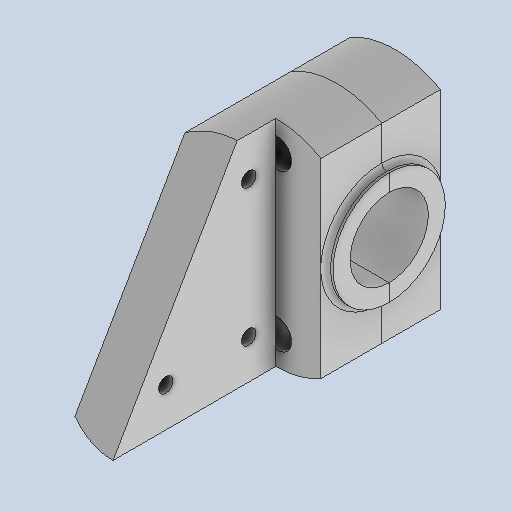
# Autodesk Inventor part: 1042
Saved by Autodesk Inventor 2025.1 (Build 291241000, 241)
## iProperties
Created: 2024-06-10
Part Number: 1042
Material: Generisch
Document SubType Name: Modeling
Designer: ffogue
Density: 1 g/cm^3
Appearance: Vorgabe
Author: ffogue
Autodesk Inventor part; units mm, degrees
note: some values were not read from the file. Chosen so that the rebuilt part matches the saved one: direction of "Bohrung4"; direction of "Bohrung11"; direction of "Bohrung12".
sketch "Skizze1" plane through (0, 0, 0) normal (0, 1, 0) x (-1, 0, 0)
  line L0 (9.25, 16.0215) -> (9.25, -23.0215)
  line L1 (-9.25, 16.0215) -> (-9.25, -23.0215)
  arc A0 (-9.25, -23.0215) -> (9.25, -23.0215) centre (0, -7) ccw
  arc A1 (9.25, 16.0215) -> (-9.25, 16.0215) centre (0, 0) ccw
  line L2 (9.25, -3.5) -> (-9.25, -3.5) construction
  line L3 (0, 18.5) -> (0, -26.5698) construction
  point P0 (0, -25.5)
  dimension "d1" = 18.5
  dimension "d2" = 44
  dimension "d3" = 18.5
  constraints: 8 end point, 6 point on circle, 2 centre point, 2 midpoint, 2 vertical, 1 coincident, 1 parallel, 1 symmetric about line, 1 other
  measures "d1" distance between parallel lines of L1 L0
  measures "d2" distance of point (0, -25.5) L3.start
  measures "d3" radius of A0
extrude "Extrusion1" add sketch "Skizze1" along normal blind 57.8
sketch "Skizze2" plane through (9.25, 0, 16.0215) normal (1, 0, 0) x (0, 0, -1)
  line L0 (0, 0) -> (-2.4785, 0) projected
  line L1 (41.5215, 0) -> (41.5215, 57.8) projected
  line L2 (0, 0) -> (39.0429, 0) projected
  line L3 (41.5215, 0) -> (39.0429, 0) projected
  line L4 (-2.4785, 0) -> (-2.4785, 57.8) projected
  line L5 (41.5215, 0) -> (-2.4785, 25.4034)
  point P0 (16.0215, 0)
  dimension "d143" = 60
  constraints: 2 end point, 1 point on line
  measures "d143" angle of L4 L5
extrude "Extrusion2" cut sketch "Skizze2" against normal up to surface (18.5 mm away)
ref_plane "Arbeitsebene1" through (0, 45.8, 0) normal (0, 1, 0) x (-1, 0, 0)
sketch "Skizze8" plane through (-9.25, 57.8, -23.0215) normal (-1, 0, 0) x (0, 0, 1)
  circle A0 centre (19.5215, -12) radius 11.5
  line L0 (0, 0) -> (39.0429, 0) projected
  point P0 (23.0215, -57.8)
  point P1 (19.5215, 0)
  dimension "d40" = 23
  dimension "d41" = 12
  constraints: 1 centre point, 1 midpoint, 1 vertical alignment
  measures "d40" diameter of A0
  measures "d41" distance from line of L0 A0.centre
extrude "Extrusion5" add sketch "Skizze8" along normal mid plane 1.5
sketch "Skizze9" plane through (9.25, 57.8, 16.0215) normal (1, 0, 0) x (0, 0, -1)
  circle A0 centre (19.5215, -12) radius 11.5
  line L0 (0, 0) -> (39.0429, 0) projected
  point P0 (16.0215, -57.8)
  point P1 (19.5215, 0)
  dimension "d44" = 23
  dimension "d45" = 12
  constraints: 1 centre point, 1 midpoint, 1 vertical alignment
  measures "d44" diameter of A0
  measures "d45" distance from line of A0.centre L0
extrude "Extrusion6" add sketch "Skizze9" along normal blind 1.5
sketch "Skizze10" plane through (10.75, 45.8, -3.5) normal (1, 0, 0) x (0, 0, -1)
  circle A0 centre (0, 0) radius 11.5 projected
  point P0 (-3.5, -45.8)
  constraints: 1 coincident
hole "Bohrung4" at (10.75, 45.8, -3.5) direction (-1, 0, 0) diameter 16 depth 20.75
ref_plane "Arbeitsebene2" through (0, 45.8, 0) normal (0, 1, 0) x (-1, 0, 0)
split_face "Trennen2"
sketch "Skizze11" plane through (0, 57.8, 0) normal (0, 1, 0) x (1, 0, 0)
  line L0 (0, 0) -> (5.4139, 0) construction
  arc A0 (-9.25, -16.0215) -> (9.25, -16.0215) centre (0, 0) ccw projected
  line L1 (0, -18.5) -> (0, 25.5) construction
  arc A1 (9.25, 23.0215) -> (-9.25, 23.0215) centre (0, 7) ccw projected
  point P0 (0, -12.5)
  point P1 (0, 19.5)
  point P2 (0, 3.5)
  dimension "d67" = 16
  dimension "d68" = 32
  constraints: 4 end point, 2 point on circle, 2 vertical alignment, 1 horizontal, 1 midpoint, 1 vertical
  measures "d67" distance of point (0, 3.5) point (0, -12.5)
  measures "d68" distance of point (0, 19.5) point (0, -12.5)
ref_plane "Arbeitsebene3" through (0, 0, 0) normal (1, 0, 0) x (0, 1, 0)
fillet "Rundung1" radius 1 2 edges at (9.25, 45.8, 8) (-9.25, 45.8, -15)
sketch "Skizze17" plane through (0, 0, 0) normal (1, 0, 0) x (0, 1, 0)
  line L0 (0, -25.5) -> (45.8, -25.5) projected
  arc A0 (45.8, -11.5) -> (45.8, 4.5) centre (45.8, -3.5) ccw projected
  arc A1 (45.8, 4.5) -> (45.8, -11.5) centre (45.8, -3.5) ccw projected
  arc A2 (45.8, 4.5) -> (45.8, -11.5) centre (45.8, -3.5) ccw projected
  line L1 (57.8, -0.1152) -> (57.8, 16.0215) projected
  point P0 (0, 0)
  point P1 (68.19, 2.5)
  dimension "d112" = 10.39
  dimension "d113" = 6
  measures "d112" distance from line of L1 point (68.19, 2.5)
  measures "d113" vertical distance of A0.centre point (68.19, 2.5)
ref_plane "Arbeitsebene8" through (0, 0, 19) normal (0, 0, 1) x (1, 0, 0)
sketch "Skizze22" plane through (0, 0, 19) normal (0, 0, 1) x (1, 0, 0)
  line L0 (-9.25, 45.8) -> (-9.25, 33.3318) projected
  line L1 (0, 0) -> (9.5, 0)
  line L2 (9.5, 0) -> (9.5, 33.3318)
  line L3 (9.5, 33.3318) -> (0, 33.3318)
  line L4 (0, 33.3318) -> (0, 0)
  dimension "d125" = 9.5
  constraints: 8 end point, 2 parallel, 1 horizontal, 1 horizontal alignment, 1 perpendicular
  measures "d125" distance between parallel lines of L2 L4
extrude "Extrusion8" cut sketch "Skizze22" against normal through all
sketch "Skizze25" plane through (-9.25, 1.431, -23.0215) normal (-1, 0, 0) x (0, 0, 1)
  line L0 (-2.4785, 31.9008) -> (-2.4785, -1.431) projected
  arc A0 (11.5215, 44.369) -> (27.5215, 44.369) centre (19.5215, 44.369) ccw projected
  arc A1 (27.5215, 44.369) -> (11.5215, 44.369) centre (19.5215, 44.369) ccw projected
  point P0 (23.0215, -1.431)
  point P1 (5.5215, 9.369)
  point P2 (5.5215, 26.369)
  point P3 (33.5215, 26.369)
  dimension "d144" = 10.8
  dimension "d145" = 14
  dimension "d146" = 17
  dimension "d147" = 14
  constraints: 1 horizontal alignment, 1 vertical alignment
  measures "d144" vertical distance of L0.end point (5.521, 9.369)
  measures "d145" horizontal distance of A0.centre point (5.521, 9.369)
  measures "d146" distance of point (5.521, 9.369) point (5.521, 26.369)
  measures "d147" horizontal distance of A0.centre point (33.521, 26.369)
hole "Bohrung11" at (-9.25, 10.8, -17.5) at (-9.25, 27.8, -17.5) at (-9.25, 27.8, 10.5) direction (1, 0, 0) diameter 3 depth 9.25 countersink diameter 5 countersink angle 90
sketch "Skizze26" plane through (0, 57.8, 0) normal (0, 1, 0) x (1, 0, 0)
  line L0 (0, 25.5) -> (0, -18.5) projected
  line L1 (-9.25, 23.0215) -> (-9.25, 6.8848) projected
  line L2 (-9.25, 0.1152) -> (-9.25, -16.0215) projected
  line L3 (9.25, 7) -> (9.25, 23.0215) projected
  line L4 (9.25, -16.0215) -> (9.25, 0) projected
  arc A0 (9.25, 23.0215) -> (-9.25, 23.0215) centre (0, 7) ccw projected
  arc A1 (-9.25, -16.0215) -> (9.25, -16.0215) centre (0, 0) ccw projected
  point P0 (0.25, 19.5)
  point P1 (0.25, -12.5)
  point P2 (0, 25.5)
  point P3 (0, -18.5)
  dimension "d155" = 9.5
  dimension "d156" = 9.5
  dimension "d157" = 6
  dimension "d158" = 6
  constraints: 2 point on circle, 2 vertical alignment
  measures "d155" distance from line of L1 point (0.25, 19.5)
  measures "d156" distance from line of L2 point (0.25, -12.5)
  measures "d157" vertical distance of point (0, 25.5) point (0.25, 19.5)
  measures "d158" vertical distance of point (0, -18.5) point (0.25, -12.5)
hole "Bohrung12" at (0.25, 57.8, 12.5) at (0.25, 57.8, -19.5) direction (0, -1, 0) diameter 6 depth 24.4682
